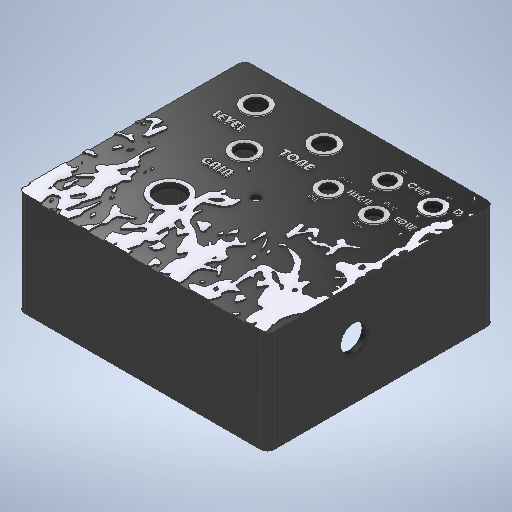
# Autodesk Inventor part: obudowa
Saved by Autodesk Inventor 2025 (Build 290162000, 162)
## iProperties
Created: 2026-04-02
Part Number: obudowa
Material: Ogólny
Document SubType Name: Modeling
Designer: zzapa
Density: 1 g/cm^3
Appearance: Domyślna
Author: zzapa
Autodesk Inventor part; units mm, degrees
(part 1 of 5)
ref_plane "YZ Plane" through (0, 0, 0) normal (1, 0, 0) x (0, 1, 0)
ref_plane "XZ Plane" through (0, 0, 0) normal (0, 1, 0) x (-1, 0, 0)
ref_plane "XY Plane" through (0, 0, 0) normal (0, 0, 1) x (1, 0, 0)
sketch "Szkic1" plane through (0, 0, 0) normal (0, 1, 0) x (-1, 0, 0)
  line L0 (110, -100) -> (0, -100)
  line L1 (0, -100) -> (0, 0)
  line L2 (0, 0) -> (110, 0)
  line L3 (110, 0) -> (110, -100)
  dimension "d0" = 100
  dimension "d1" = 110
  constraints: 8 end point, 2 parallel, 1 coincident, 1 horizontal, 1 perpendicular
  measures "d0" distance of L2.end L0.start
  measures "d1" distance of L0.start L0.end
extrude "Gabaryt" add sketch "Szkic1" along normal blind 45
ref_plane "Konstrukcja wycięcia" through (0, 43, 0) normal (0, 1, 0) x (1, 0, 0)
sketch "Szkic2" plane through (0, 0, 0) normal (0, -1, 0) x (1, 0, 0)
  line L0 (-110, 0) -> (0, 0) projected
  line L1 (-110, -100) -> (-110, 0) projected
  line L2 (0, -100) -> (-110, -100) projected
  line L3 (0, 0) -> (0, -100) projected
  line L4 (-2, -98) -> (-108, -98)
  line L5 (-108, -98) -> (-108, -2)
  line L6 (-108, -2) -> (-2, -2)
  line L7 (-2, -2) -> (-2, -98)
  dimension "d4" = 2
  constraints: 8 end point, 3 other
  measures "d4" distance between parallel lines of L3 L7
extrude "Wydrążenie" cut sketch "Szkic2" against normal up to surface (43 mm away) contours L4 L5 L6 L7
sketch "Szkic6" plane through (0, 0, 0) normal (0, -1, 0) x (1, 0, 0)
  line L0 (-110, 0) -> (0, 0) projected
  line L1 (-8, -8) -> (0, -8)
  line L2 (0, -8) -> (0, 0)
  line L3 (0, 0) -> (-8, 0)
  line L4 (-8, 0) -> (-8, -8)
  line L5 (0, 0) -> (0, -100) projected
  line L6 (0, -100) -> (-110, -100) projected
  line L7 (-110, -100) -> (-110, 0) projected
  line L8 (0, 0) -> (0, -100) projected
  line L9 (0, -50) -> (-110, -50)
  line L10 (-55, 0) -> (-55, -100)
  line L11 (-102, -8) -> (-110, -8)
  line L12 (-110, -8) -> (-110, 0)
  line L13 (-110, 0) -> (-102, 0)
  line L14 (-102, 0) -> (-102, -8)
  line L15 (-8, -92) -> (0, -92)
  line L16 (0, -92) -> (0, -100)
  line L17 (0, -100) -> (-8, -100)
  line L18 (-8, -100) -> (-8, -92)
  line L19 (-102, -92) -> (-110, -92)
  line L20 (-110, -92) -> (-110, -100)
  line L21 (-110, -100) -> (-102, -100)
  line L22 (-102, -100) -> (-102, -92)
  point P0 (-102, -100)
  point P1 (-110, -92)
  point P2 (-102, 0)
  point P3 (-8, -100)
  point P4 (0, -92)
  point P5 (-8, 0)
  dimension "d16" = 8
  dimension "d17" = 8
  constraints: 36 end point, 9 symmetric about line, 4 midpoint, 2 parallel, 1 horizontal, 1 perpendicular
  measures "d16" distance of L1.start L1.end
  measures "d17" distance of L3.end L1.start
extrude "Materiał na insert" add sketch "Szkic6" against normal up to surface (43 mm away) contours L0 L14 L11 L7 | L0 L2 L1 L4 | L19 L22 L6 L7 | L5 L6 L18 L15
sketch "Szkic7" plane through (0, 0, 0) normal (0, -1, 0) x (1, 0, 0)
  line L0 (0, 0) -> (0, -100) projected
  line L1 (0, -50) -> (-110, -50)
  line L2 (-110, -100) -> (-110, 0) projected
  line L3 (0, -100) -> (-110, -100) projected
  line L4 (-55, -100) -> (-55, 0)
  line L5 (-110, 0) -> (0, 0) projected
  point P0 (-4, -4)
  point P1 (-106, -4)
  point P2 (-4, -96)
  point P3 (-106, -96)
  dimension "d20" = 4
  dimension "d21" = 4
  constraints: 4 end point, 4 midpoint, 3 symmetric about line
  measures "d20" horizontal distance of L0.start point (-4, -4)
  measures "d21" horizontal distance of point (-4, -4) L0.start
hole "Otwory montażowe" at (-4, 0, -4) at (-106, 0, -4) at (-4, 0, -96) at (-106, 0, -96) direction (0, 1, 0) diameter 2.4 depth 5.5
fillet "Zaokrąglenie1" radius 3 4 edges at (-110, 22.5, 0) (0, 22.5, 0) (0, 22.5, -100) (-110, 22.5, -100)
sketch "Szkic8" plane through (-110, 0, -97) normal (-1, 0, 0) x (0, 0, 1)
  line L0 (-3, 45) -> (-3, 0) projected
  line L1 (0, 0) -> (94, 0) projected
  line L2 (0, 0) -> (-3, 0) projected
  line L3 (97, 0) -> (97, 45) projected
  point P0 (42, 25)
  dimension "d30" = 25
  dimension "d39" = 55
  measures "d30" distance from line of L1 point (42, 25)
  measures "d39" distance from line of L3 point (42, 25)
hole "JACK 1" at (-110, 25, -55) direction (1, 0, 0) diameter 11.5 depth 2
sketch "Szkic9" plane through (0, 0, -3) normal (1, 0, 0) x (0, 0, -1)
  line L0 (0, 0) -> (94, 0) projected
  line L1 (-3, 45) -> (-3, 0) projected
  point P0 (35, 25)
  dimension "d40" = 25
  dimension "d41" = 38
  measures "d40" distance from line of L0 point (35, 25)
  measures "d41" distance from line of point (35, 25) L1
hole "JACK 2" at (0, 25, -38) direction (-1, 0, 0) diameter 11.5 end up to face face through (-2, 14.3333, -64) facing (-1, 0, 0)
sketch "Szkic16" plane through (0, 45, 0) normal (0, 1, 0) x (1, 0, 0)
  line L0 (-138.1067, 105.9838) -> (23.8181, 105.9838)
  line L1 (23.8181, 105.9838) -> (23.8181, 34.811)
  line L2 (23.8181, 34.811) -> (23.0109, 35.22)
  line L3 (23.0109, 35.22) -> (22.3629, 35.8693)
  line L4 (22.3629, 35.8693) -> (21.7155, 38.0761)
  line L5 (21.7155, 38.0761) -> (20.9077, 40.2349)
  line L6 (20.9077, 40.2349) -> (21.2638, 40.857)
  line L7 (21.2638, 40.857) -> (21.4369, 41.5579)
  line L8 (21.4369, 41.5579) -> (21.3046, 46.1881)
  line L9 (21.3046, 46.1881) -> (20.2689, 48.7465)
  line L10 (20.2689, 48.7465) -> (19.0556, 51.2151)
  line L11 (19.0556, 51.2151) -> (19.3469, 52.5366)
  line L12 (19.3469, 52.5366) -> (19.4525, 53.861)
  line L13 (19.4525, 53.861) -> (19.1879, 54.3901)
  line L14 (19.1879, 54.3901) -> (18.0583, 53.9543)
  line L15 (18.0583, 53.9543) -> (17.1306, 54.0295)
  line L16 (17.1306, 54.0295) -> (16.4047, 54.6158)
  line L17 (16.4047, 54.6158) -> (15.8806, 55.7131)
  line L18 (15.8806, 55.7131) -> (16.2764, 57.0344)
  line L19 (16.2764, 57.0344) -> (16.939, 58.2266)
  line L20 (16.939, 58.2266) -> (19.3202, 58.6235)
  line L21 (19.3202, 58.6235) -> (19.5271, 59.3328)
  line L22 (19.5271, 59.3328) -> (19.53, 60.0102)
  line L23 (19.53, 60.0102) -> (19.3287, 60.6557)
  line L24 (19.3287, 60.6557) -> (18.9233, 61.2693)
  line L25 (18.9233, 61.2693) -> (17.8565, 60.6698)
  line L26 (17.8565, 60.6698) -> (16.6744, 60.3433)
  line L27 (16.6744, 60.3433) -> (16.2775, 58.6235)
  line L28 (16.2775, 58.6235) -> (15.4838, 58.0943)
  line L29 (15.4838, 58.0943) -> (15.0261, 58.2056)
  line L30 (15.0261, 58.2056) -> (14.631, 58.1325)
  line L31 (14.631, 58.1325) -> (14.2984, 57.8749)
  line L32 (14.2984, 57.8749) -> (14.0286, 57.4328)
  line L33 (14.0286, 57.4328) -> (12.4411, 57.3005)
  line L34 (12.4411, 57.3005) -> (10.8536, 57.4328)
  line L35 (10.8536, 57.4328) -> (9.5248, 58.7629)
  line L36 (9.5248, 58.7629) -> (8.4723, 60.3433)
  line L37 (8.4723, 60.3433) -> (1.4609, 64.1797)
  line L38 (1.4609, 64.1797) -> (-0.1266, 67.3547)
  line L39 (-0.1266, 67.3547) -> (-0.1433, 69.3393)
  line L40 (-0.1433, 69.3393) -> (0.0057, 71.3234)
  line L41 (0.0057, 71.3234) -> (-0.7881, 71.3234)
  line L42 (-0.7881, 71.3234) -> (-1.1487, 69.1464)
  line L43 (-1.1487, 69.1464) -> (-1.3629, 68.6021)
  line L44 (-1.3629, 68.6021) -> (-1.5997, 68.4207)
  line L45 (-1.5997, 68.4207) -> (-1.859, 68.6021)
  line L46 (-1.859, 68.6021) -> (-2.1409, 69.1464)
  line L47 (-2.1409, 69.1464) -> (-2.7725, 71.3234)
  line L48 (-2.7725, 71.3234) -> (-2.9048, 72.7787)
  line L49 (-2.9048, 72.7787) -> (-2.7725, 74.2339)
  line L50 (-2.7725, 74.2339) -> (2.1223, 76.4828)
  line L51 (2.1223, 76.4828) -> (3.588, 77.6838)
  line L52 (3.588, 77.6838) -> (4.6359, 79.2609)
  line L53 (4.6359, 79.2609) -> (4.7682, 81.6422)
  line L54 (4.7682, 81.6422) -> (4.6359, 84.0234)
  line L55 (4.6359, 84.0234) -> (3.1196, 87.6571)
  line L56 (3.1196, 87.6571) -> (1.3286, 91.1672)
  line L57 (1.3286, 91.1672) -> (0.4638, 91.3959)
  line L58 (0.4638, 91.3959) -> (-0.2654, 91.2958)
  line L59 (-0.2654, 91.2958) -> (-0.8591, 90.8667)
  line L60 (-0.8591, 90.8667) -> (-1.3173, 90.1088)
  line L61 (-1.3173, 90.1088) -> (-0.6682, 89.4152)
  line L62 (-0.6682, 89.4152) -> (0.2702, 89.1828)
  line L63 (0.2702, 89.1828) -> (0.7636, 88.4018)
  line L64 (0.7636, 88.4018) -> (1.1044, 87.5683)
  line L65 (1.1044, 87.5683) -> (1.2928, 86.682)
  line L66 (1.2928, 86.682) -> (1.3286, 85.7432)
  line L67 (1.3286, 85.7432) -> (1.1916, 84.5366)
  line L68 (1.1916, 84.5366) -> (0.9519, 83.618)
  line L69 (0.9519, 83.618) -> (0.6097, 82.9875)
  line L70 (0.6097, 82.9875) -> (0.1649, 82.645)
  line L71 (0.1649, 82.645) -> (-0.3824, 82.5906)
  line L72 (-0.3824, 82.5906) -> (-1.0324, 82.8243)
  line L73 (-1.0324, 82.8243) -> (-1.785, 83.346)
  line L74 (-1.785, 83.346) -> (-2.6402, 84.1557)
  line L75 (-2.6402, 84.1557) -> (-3.4339, 84.288)
  line L76 (-3.4339, 84.288) -> (-3.408, 82.9177)
  line L77 (-3.408, 82.9177) -> (-3.7742, 81.7554)
  line L78 (-3.7742, 81.7554) -> (-4.5325, 80.8011)
  line L79 (-4.5325, 80.8011) -> (-5.6829, 80.0547)
  line L80 (-5.6829, 80.0547) -> (-5.9576, 79.4144)
  line L81 (-5.9576, 79.4144) -> (-6.0271, 78.782)
  line L82 (-6.0271, 78.782) -> (-5.8915, 78.1577)
  line L83 (-5.8915, 78.1577) -> (-5.5506, 77.5411)
  line L84 (-5.5506, 77.5411) -> (-6.0348, 75.915)
  line L85 (-6.0348, 75.915) -> (-6.3443, 74.2339)
  line L86 (-6.3443, 74.2339) -> (-6.0798, 72.9109)
  line L87 (-6.0798, 72.9109) -> (-6.3443, 71.588)
  line L88 (-6.3443, 71.588) -> (-3.1693, 63.7828)
  line L89 (-3.1693, 63.7828) -> (-3.5662, 62.3276)
  line L90 (-3.5662, 62.3276) -> (-4.1521, 61.7435)
  line L91 (-4.1521, 61.7435) -> (-4.4922, 61.0047)
  line L92 (-4.4922, 61.0047) -> (-3.5983, 56.4054)
  line L93 (-3.5983, 56.4054) -> (-3.3753, 54.0825)
  line L94 (-3.3753, 54.0825) -> (-3.3016, 51.7443)
  line L95 (-3.3016, 51.7443) -> (-4.0954, 50.1568)
  line L96 (-4.0954, 50.1568) -> (-7.0058, 47.7756)
  line L97 (-7.0058, 47.7756) -> (-7.535, 45.3943)
  line L98 (-7.535, 45.3943) -> (-9.1611, 44.8525)
  line L99 (-9.1611, 44.8525) -> (-10.8422, 44.4683)
  line L100 (-10.8422, 44.4683) -> (-11.3602, 43.7585)
  line L101 (-11.3602, 43.7585) -> (-11.6431, 43.0148)
  line L102 (-11.6431, 43.0148) -> (-11.6909, 42.2371)
  line L103 (-11.6909, 42.2371) -> (-11.5037, 41.4256)
  line L104 (-11.5037, 41.4256) -> (-10.3341, 40.2553)
  line L105 (-10.3341, 40.2553) -> (-8.9902, 39.3089)
  line L106 (-8.9902, 39.3089) -> (-8.0825, 39.6923)
  line L107 (-8.0825, 39.6923) -> (-7.1846, 39.8201)
  line L108 (-7.1846, 39.8201) -> (-6.2965, 39.6923)
  line L109 (-6.2965, 39.6923) -> (-5.4183, 39.3089)
  line L110 (-5.4183, 39.3089) -> (-5.1545, 38.9347)
  line L111 (-5.1545, 38.9347) -> (-5.0887, 38.5675)
  line L112 (-5.0887, 38.5675) -> (-5.2207, 38.2072)
  line L113 (-5.2207, 38.2072) -> (-5.5506, 37.8537)
  line L114 (-5.5506, 37.8537) -> (-6.457, 37.4644)
  line L115 (-6.457, 37.4644) -> (-7.2704, 36.9277)
  line L116 (-7.2704, 36.9277) -> (-7.3598, 36.574)
  line L117 (-7.3598, 36.574) -> (-7.1381, 36.2662)
  line L118 (-7.1381, 36.2662) -> (-6.6089, 36.1338)
  line L119 (-6.6089, 36.1338) -> (-6.0797, 36.2662)
  line L120 (-6.0797, 36.2662) -> (-5.3543, 36.8938)
  line L121 (-5.3543, 36.8938) -> (-4.4922, 37.3245)
  line L122 (-4.4922, 37.3245) -> (-4.2715, 38.0841)
  line L123 (-4.2715, 38.0841) -> (-4.2277, 38.7797)
  line L124 (-4.2277, 38.7797) -> (-2.6402, 37.7214)
  line L125 (-2.6402, 37.7214) -> (-2.0611, 35.7499)
  line L126 (-2.0611, 35.7499) -> (-1.7141, 33.7527)
  line L127 (-1.7141, 33.7527) -> (-2.2126, 34.1473)
  line L128 (-2.2126, 34.1473) -> (-2.6654, 34.2568)
  line L129 (-2.6654, 34.2568) -> (-3.0725, 34.0812)
  line L130 (-3.0725, 34.0812) -> (-3.4339, 33.6204)
  line L131 (-3.4339, 33.6204) -> (-3.1209, 33.0089)
  line L132 (-3.1209, 33.0089) -> (-2.7299, 32.7389)
  line L133 (-2.7299, 32.7389) -> (-2.261, 32.8104)
  line L134 (-2.261, 32.8104) -> (-1.7141, 33.2235)
  line L135 (-1.7141, 33.2235) -> (-1.4495, 32.9589)
  line L136 (-1.4495, 32.9589) -> (-1.7141, 30.0485)
  line L137 (-1.7141, 30.0485) -> (-0.1266, 29.2548)
  line L138 (-0.1266, 29.2548) -> (0.0057, 28.461)
  line L139 (0.0057, 28.461) -> (-0.1266, 27.6673)
  line L140 (-0.1266, 27.6673) -> (-1.9787, 27.4027)
  line L141 (-1.9787, 27.4027) -> (-2.4802, 26.1616)
  line L142 (-2.4802, 26.1616) -> (-3.1693, 25.0214)
  line L143 (-3.1693, 25.0214) -> (-2.9048, 24.4923)
  line L144 (-2.9048, 24.4923) -> (-3.1693, 23.9631)
  line L145 (-3.1693, 23.9631) -> (-6.0797, 23.8308)
  line L146 (-6.0797, 23.8308) -> (-6.6591, 23.3711)
  line L147 (-6.6591, 23.3711) -> (-7.2491, 23.2178)
  line L148 (-7.2491, 23.2178) -> (-7.8498, 23.3711)
  line L149 (-7.8498, 23.3711) -> (-8.461, 23.8308)
  line L150 (-8.461, 23.8308) -> (-9.1787, 24.6043)
  line L151 (-9.1787, 24.6043) -> (-9.6516, 25.5506)
  line L152 (-9.6516, 25.5506) -> (-10.0048, 27.4854)
  line L153 (-10.0048, 27.4854) -> (-10.0485, 29.387)
  line L154 (-10.0485, 29.387) -> (-10.9894, 29.4565)
  line L155 (-10.9894, 29.4565) -> (-11.6999, 29.1931)
  line L156 (-11.6999, 29.1931) -> (-12.18, 28.5967)
  line L157 (-12.18, 28.5967) -> (-12.4297, 27.6673)
  line L158 (-12.4297, 27.6673) -> (-12.8266, 27.2703)
  line L159 (-12.8266, 27.2703) -> (-13.2235, 27.138)
  line L160 (-13.2235, 27.138) -> (-13.6204, 27.2703)
  line L161 (-13.6204, 27.2703) -> (-14.0172, 27.6673)
  line L162 (-14.0172, 27.6673) -> (-15.0756, 29.387)
  line L163 (-15.0756, 29.387) -> (-15.8613, 29.6807)
  line L164 (-15.8613, 29.6807) -> (-16.4539, 30.1534)
  line L165 (-16.4539, 30.1534) -> (-16.8535, 30.8052)
  line L166 (-16.8535, 30.8052) -> (-17.0599, 31.636)
  line L167 (-17.0599, 31.636) -> (-20.8964, 36.0016)
  line L168 (-20.8964, 36.0016) -> (-25.3943, 37.3245)
  line L169 (-25.3943, 37.3245) -> (-26.8515, 37.5331)
  line L170 (-26.8515, 37.5331) -> (-28.3047, 37.5891)
  line L171 (-28.3047, 37.5891) -> (-28.5692, 37.3245)
  line L172 (-28.5692, 37.3245) -> (-28.3047, 37.06)
  line L173 (-28.3047, 37.06) -> (-24.5793, 35.33)
  line L174 (-24.5793, 35.33) -> (-21.161, 33.0912)
  line L175 (-21.161, 33.0912) -> (-19.5551, 30.806)
  line L176 (-19.5551, 30.806) -> (-18.2506, 28.3287)
  line L177 (-18.2506, 28.3287) -> (-19.1787, 27.2531)
  line L178 (-19.1787, 27.2531) -> (-20.2818, 26.5197)
  line L179 (-20.2818, 26.5197) -> (-21.5599, 26.1286)
  line L180 (-21.5599, 26.1286) -> (-23.0131, 26.0798)
  line L181 (-23.0131, 26.0798) -> (-25.1306, 26.2504)
  line L182 (-25.1306, 26.2504) -> (-27.2464, 25.9475)
  line L183 (-27.2464, 25.9475) -> (-27.6953, 25.1448)
  line L184 (-27.6953, 25.1448) -> (-27.889, 24.3261)
  line L185 (-27.889, 24.3261) -> (-27.8275, 23.4912)
  line L186 (-27.8275, 23.4912) -> (-27.511, 22.6402)
  line L187 (-27.511, 22.6402) -> (-28.3047, 20.3912)
  line L188 (-28.3047, 20.3912) -> (-27.2464, 13.2475)
  line L189 (-27.2464, 13.2475) -> (-27.511, 11.66)
  line L190 (-27.511, 11.66) -> (-27.7756, 11.5277)
  line L191 (-27.7756, 11.5277) -> (-28.0306, 12.165)
  line L192 (-28.0306, 12.165) -> (-28.0401, 12.8506)
  line L193 (-28.0401, 12.8506) -> (-28.8807, 12.6734)
  line L194 (-28.8807, 12.6734) -> (-29.4953, 12.0569)
  line L195 (-29.4953, 12.0569) -> (-30.8183, 9.6756)
  line L196 (-30.8183, 9.6756) -> (-31.612, 4.6485)
  line L197 (-31.612, 4.6485) -> (-32.2735, 3.9871)
  line L198 (-32.2735, 3.9871) -> (-34.1565, 3.5577)
  line L199 (-34.1565, 3.5577) -> (-35.9776, 2.9287)
  line L200 (-35.9776, 2.9287) -> (-36.2243, 2.2225)
  line L201 (-36.2243, 2.2225) -> (-36.1099, 1.4735)
  line L202 (-36.1099, 1.4735) -> (-34.1255, -0.2463)
  line L203 (-34.1255, -0.2463) -> (-31.4797, -0.2463)
  line L204 (-31.4797, -0.2463) -> (-30.7853, -1.0092)
  line L205 (-30.7853, -1.0092) -> (-30.4214, -1.966)
  line L206 (-30.4214, -1.966) -> (-39.1526, -1.966)
  line L207 (-39.1526, -1.966) -> (-38.8027, 0.0962)
  line L208 (-38.8027, 0.0962) -> (-38.7963, 2.1506)
  line L209 (-38.7963, 2.1506) -> (-39.1334, 4.1972)
  line L210 (-39.1334, 4.1972) -> (-39.8141, 6.236)
  line L211 (-39.8141, 6.236) -> (-39.9464, 7.8235)
  line L212 (-39.9464, 7.8235) -> (-39.8141, 9.411)
  line L213 (-39.8141, 9.411) -> (-39.4254, 10.189)
  line L214 (-39.4254, 10.189) -> (-38.888, 10.8662)
  line L215 (-38.888, 10.8662) -> (-37.0454, 11.9188)
  line L216 (-37.0454, 11.9188) -> (-35.3162, 13.1152)
  line L217 (-35.3162, 13.1152) -> (-34.2564, 12.3146)
  line L218 (-34.2564, 12.3146) -> (-33.4641, 11.2631)
  line L219 (-33.4641, 11.2631) -> (-33.0886, 11.3881)
  line L220 (-33.0886, 11.3881) -> (-32.8026, 11.66)
  line L221 (-32.8026, 11.66) -> (-34.1364, 13.789)
  line L222 (-34.1364, 13.789) -> (-35.713, 15.761)
  line L223 (-35.713, 15.761) -> (-36.9086, 16.0817)
  line L224 (-36.9086, 16.0817) -> (-38.0943, 16.0256)
  line L225 (-38.0943, 16.0256) -> (-37.3997, 15.6813)
  line L226 (-37.3997, 15.6813) -> (-36.8815, 15.2137)
  line L227 (-36.8815, 15.2137) -> (-36.5397, 14.623)
  line L228 (-36.5397, 14.623) -> (-36.3745, 13.9089)
  line L229 (-36.3745, 13.9089) -> (-36.906, 13.4522)
  line L230 (-36.906, 13.4522) -> (-37.48, 13.2118)
  line L231 (-37.48, 13.2118) -> (-38.0966, 13.1876)
  line L232 (-38.0966, 13.1876) -> (-38.7557, 13.3798)
  line L233 (-38.7557, 13.3798) -> (-39.4851, 12.7013)
  line L234 (-39.4851, 12.7013) -> (-40.4755, 12.586)
  line L235 (-40.4755, 12.586) -> (-40.2419, 14.0455)
  line L236 (-40.2419, 14.0455) -> (-39.7451, 15.3698)
  line L237 (-39.7451, 15.3698) -> (-38.9851, 16.5591)
  line L238 (-38.9851, 16.5591) -> (-37.962, 17.6131)
  line L239 (-37.962, 17.6131) -> (-37.5934, 19.1841)
  line L240 (-37.5934, 19.1841) -> (-37.8297, 20.7881)
  line L241 (-37.8297, 20.7881) -> (-39.4129, 21.5569)
  line L242 (-39.4129, 21.5569) -> (-40.5863, 22.3706)
  line L243 (-40.5863, 22.3706) -> (-41.3499, 23.2292)
  line L244 (-41.3499, 23.2292) -> (-41.7036, 24.1328)
  line L245 (-41.7036, 24.1328) -> (-41.6475, 25.0813)
  line L246 (-41.6475, 25.0813) -> (-41.1816, 26.0747)
  line L247 (-41.1816, 26.0747) -> (-40.3059, 27.1131)
  line L248 (-40.3059, 27.1131) -> (-39.0203, 28.1964)
  line L249 (-39.0203, 28.1964) -> (-38.6861, 29.0417)
  line L250 (-38.6861, 29.0417) -> (-38.729, 29.6982)
  line L251 (-38.729, 29.6982) -> (-39.1491, 30.1661)
  line L252 (-39.1491, 30.1661) -> (-39.9464, 30.4454)
  line L253 (-39.9464, 30.4454) -> (-40.3009, 29.6426)
  line L254 (-40.3009, 29.6426) -> (-40.8724, 28.9902)
  line L255 (-40.8724, 28.9902) -> (-41.9146, 29.5033)
  line L256 (-41.9146, 29.5033) -> (-42.8568, 30.1808)
  line L257 (-42.8568, 30.1808) -> (-43.5366, 30.306)
  line L258 (-43.5366, 30.306) -> (-44.1797, 30.0485)
  line L259 (-44.1797, 30.0485) -> (-43.2841, 28.6643)
  line L260 (-43.2841, 28.6643) -> (-43.1264, 28.0537)
  line L261 (-43.1264, 28.0537) -> (-43.162, 27.4974)
  line L262 (-43.162, 27.4974) -> (-43.391, 26.9954)
  line L263 (-43.391, 26.9954) -> (-43.8134, 26.5477)
  line L264 (-43.8134, 26.5477) -> (-45.238, 25.8152)
  line L265 (-45.238, 25.8152) -> (-45.8113, 25.9916)
  line L266 (-45.8113, 25.9916) -> (-46.2964, 26.3443)
  line L267 (-46.2964, 26.3443) -> (-46.8255, 25.5506)
  line L268 (-46.8255, 25.5506) -> (-45.7672, 22.5079)
  line L269 (-45.7672, 22.5079) -> (-45.9219, 22.0886)
  line L270 (-45.9219, 22.0886) -> (-46.2964, 21.8464)
  line L271 (-46.2964, 21.8464) -> (-47.7516, 22.9048)
  line L272 (-47.7516, 22.9048) -> (-48.1484, 22.5079)
  line L273 (-48.1484, 22.5079) -> (-46.8255, 20.7881)
  line L274 (-46.8255, 20.7881) -> (-47.3547, 19.4652)
  line L275 (-47.3547, 19.4652) -> (-48.9521, 19.2457)
  line L276 (-48.9521, 19.2457) -> (-50.5297, 19.5975)
  line L277 (-50.5297, 19.5975) -> (-51.946, 21.0018)
  line L278 (-51.946, 21.0018) -> (-53.4765, 22.2637)
  line L279 (-53.4765, 22.2637) -> (-55.121, 23.3831)
  line L280 (-55.121, 23.3831) -> (-56.8797, 24.36)
  line L281 (-56.8797, 24.36) -> (-58.39, 24.9104)
  line L282 (-58.39, 24.9104) -> (-59.6211, 25.7774)
  line L283 (-59.6211, 25.7774) -> (-60.5728, 26.9609)
  line L284 (-60.5728, 26.9609) -> (-61.2453, 28.461)
  line L285 (-61.2453, 28.461) -> (-61.5301, 29.4351)
  line L286 (-61.5301, 29.4351) -> (-61.6422, 30.4454)
  line L287 (-61.6422, 30.4454) -> (-61.4954, 31.704)
  line L288 (-61.4954, 31.704) -> (-61.5099, 32.9589)
  line L289 (-61.5099, 32.9589) -> (-61.9068, 33.2235)
  line L290 (-61.9068, 33.2235) -> (-62.9651, 30.3131)
  line L291 (-62.9651, 30.3131) -> (-63.7676, 31.5253)
  line L292 (-63.7676, 31.5253) -> (-64.1557, 32.9589)
  line L293 (-64.1557, 32.9589) -> (-64.3891, 34.5696)
  line L294 (-64.3891, 34.5696) -> (-64.1557, 36.1339)
  line L295 (-64.1557, 36.1339) -> (-59.2609, 38.3829)
  line L296 (-59.2609, 38.3829) -> (-58.2504, 39.0964)
  line L297 (-58.2504, 39.0964) -> (-57.4726, 39.9737)
  line L298 (-57.4726, 39.9737) -> (-56.9275, 41.0147)
  line L299 (-56.9275, 41.0147) -> (-56.6151, 42.2193)
  line L300 (-56.6151, 42.2193) -> (-56.7474, 45.1297)
  line L301 (-56.7474, 45.1297) -> (-57.3205, 45.3719)
  line L302 (-57.3205, 45.3719) -> (-57.938, 45.262)
  line L303 (-57.938, 45.262) -> (-58.6076, 44.4039)
  line L304 (-58.6076, 44.4039) -> (-59.4041, 43.9194)
  line L305 (-59.4041, 43.9194) -> (-60.3274, 43.8086)
  line L306 (-60.3274, 43.8086) -> (-61.3776, 44.0714)
  line L307 (-61.3776, 44.0714) -> (-62.4004, 43.6928)
  line L308 (-62.4004, 43.6928) -> (-63.2297, 43.0131)
  line L309 (-63.2297, 43.0131) -> (-63.4943, 43.2777)
  line L310 (-63.4943, 43.2777) -> (-63.1209, 43.7814)
  line L311 (-63.1209, 43.7814) -> (-62.9744, 44.3021)
  line L312 (-62.9744, 44.3021) -> (-63.0547, 44.8397)
  line L313 (-63.0547, 44.8397) -> (-63.362, 45.3943)
  line L314 (-63.362, 45.3943) -> (-64.0124, 45.8551)
  line L315 (-64.0124, 45.8551) -> (-64.8172, 45.9235)
  line L316 (-64.8172, 45.9235) -> (-64.9495, 44.0714)
  line L317 (-64.9495, 44.0714) -> (-67.0661, 41.4256)
  line L318 (-67.0661, 41.4256) -> (-67.7276, 35.2079)
  line L319 (-67.7276, 35.2079) -> (-67.5953, 32.4297)
  line L320 (-67.5953, 32.4297) -> (-66.4892, 30.4341)
  line L321 (-66.4892, 30.4341) -> (-65.6109, 28.3287)
  line L322 (-65.6109, 28.3287) -> (-65.8969, 28.0569)
  line L323 (-65.8969, 28.0569) -> (-66.2724, 27.9318)
  line L324 (-66.2724, 27.9318) -> (-68.0585, 28.7584)
  line L325 (-68.0585, 28.7584) -> (-69.712, 29.7839)
  line L326 (-69.712, 29.7839) -> (-70.5057, 32.9589)
  line L327 (-70.5057, 32.9589) -> (-70.7581, 32.4963)
  line L328 (-70.7581, 32.4963) -> (-70.8202, 32.0334)
  line L329 (-70.8202, 32.0334) -> (-70.692, 31.5702)
  line L330 (-70.692, 31.5702) -> (-70.3734, 31.1068)
  line L331 (-70.3734, 31.1068) -> (-70.563, 30.1469)
  line L332 (-70.563, 30.1469) -> (-70.979, 29.364)
  line L333 (-70.979, 29.364) -> (-71.6214, 28.7579)
  line L334 (-71.6214, 28.7579) -> (-72.4901, 28.3287)
  line L335 (-72.4901, 28.3287) -> (-73.6247, 27.1948)
  line L336 (-73.6247, 27.1948) -> (-74.6067, 25.9475)
  line L337 (-74.6067, 25.9475) -> (-74.2868, 25.3081)
  line L338 (-74.2868, 25.3081) -> (-74.136, 24.6539)
  line L339 (-74.136, 24.6539) -> (-74.1545, 23.9851)
  line L340 (-74.1545, 23.9851) -> (-74.3422, 23.3016)
  line L341 (-74.3422, 23.3016) -> (-74.0142, 22.7184)
  line L342 (-74.0142, 22.7184) -> (-73.5961, 22.4358)
  line L343 (-73.5961, 22.4358) -> (-73.0881, 22.4538)
  line L344 (-73.0881, 22.4538) -> (-72.4901, 22.7725)
  line L345 (-72.4901, 22.7725) -> (-70.846, 24.1135)
  line L346 (-70.846, 24.1135) -> (-70.2283, 24.3413)
  line L347 (-70.2283, 24.3413) -> (-69.7468, 24.2739)
  line L348 (-69.7468, 24.2739) -> (-69.4015, 23.9113)
  line L349 (-69.4015, 23.9113) -> (-69.1924, 23.2536)
  line L350 (-69.1924, 23.2536) -> (-69.1828, 21.0527)
  line L351 (-69.1828, 21.0527) -> (-67.9922, 17.3485)
  line L352 (-67.9922, 17.3485) -> (-68.0951, 16.9229)
  line L353 (-68.0951, 16.9229) -> (-68.3057, 16.6708)
  line L354 (-68.3057, 16.6708) -> (-68.6242, 16.5922)
  line L355 (-68.6242, 16.5922) -> (-69.0505, 16.6871)
  line L356 (-69.0505, 16.6871) -> (-69.8572, 18.8427)
  line L357 (-69.8572, 18.8427) -> (-70.5057, 21.0527)
  line L358 (-70.5057, 21.0527) -> (-71.2849, 21.0981)
  line L359 (-71.2849, 21.0981) -> (-71.7652, 20.8487)
  line L360 (-71.7652, 20.8487) -> (-71.9464, 20.3044)
  line L361 (-71.9464, 20.3044) -> (-71.8286, 19.4652)
  line L362 (-71.8286, 19.4652) -> (-70.7346, 17.8066)
  line L363 (-70.7346, 17.8066) -> (-69.4474, 16.2902)
  line L364 (-69.4474, 16.2902) -> (-69.3348, 15.2084)
  line L365 (-69.3348, 15.2084) -> (-69.5398, 14.2524)
  line L366 (-69.5398, 14.2524) -> (-70.0624, 13.4224)
  line L367 (-70.0624, 13.4224) -> (-70.9026, 12.7183)
  line L368 (-70.9026, 12.7183) -> (-72.1541, 12.3764)
  line L369 (-72.1541, 12.3764) -> (-73.4161, 12.3214)
  line L370 (-73.4161, 12.3214) -> (-73.4655, 11.1487)
  line L371 (-73.4655, 11.1487) -> (-73.3496, 10.0081)
  line L372 (-73.3496, 10.0081) -> (-73.0686, 8.8997)
  line L373 (-73.0686, 8.8997) -> (-72.6224, 7.8235)
  line L374 (-72.6224, 7.8235) -> (-71.197, 8.9175)
  line L375 (-71.197, 8.9175) -> (-69.9943, 10.1862)
  line L376 (-69.9943, 10.1862) -> (-69.0142, 11.6295)
  line L377 (-69.0142, 11.6295) -> (-68.2568, 13.2475)
  line L378 (-68.2568, 13.2475) -> (-67.4827, 13.5231)
  line L379 (-67.4827, 13.5231) -> (-66.8278, 13.4606)
  line L380 (-66.8278, 13.4606) -> (-66.2921, 13.0601)
  line L381 (-66.2921, 13.0601) -> (-65.8755, 12.3214)
  line L382 (-65.8755, 12.3214) -> (-66.4047, 11.3954)
  line L383 (-66.4047, 11.3954) -> (-67.6284, 10.6671)
  line L384 (-67.6284, 10.6671) -> (-68.4552, 9.6968)
  line L385 (-68.4552, 9.6968) -> (-68.8851, 8.4843)
  line L386 (-68.8851, 8.4843) -> (-68.9182, 7.0298)
  line L387 (-68.9182, 7.0298) -> (-69.8443, 6.1037)
  line L388 (-69.8443, 6.1037) -> (-73.1515, 4.9131)
  line L389 (-73.1515, 4.9131) -> (-72.6447, 2.0679)
  line L390 (-72.6447, 2.0679) -> (-71.564, -0.6431)
  line L391 (-71.564, -0.6431) -> (-71.4317, -1.966)
  line L392 (-71.4317, -1.966) -> (-78.3109, -1.966)
  line L393 (-78.3109, -1.966) -> (-78.6487, -0.117)
  line L394 (-78.6487, -0.117) -> (-78.7833, 1.7342)
  line L395 (-78.7833, 1.7342) -> (-78.7148, 3.5872)
  line L396 (-78.7148, 3.5872) -> (-78.4432, 5.4423)
  line L397 (-78.4432, 5.4423) -> (-77.5172, 7.0298)
  line L398 (-77.5172, 7.0298) -> (-77.9934, 9.3856)
  line L399 (-77.9934, 9.3856) -> (-77.914, 11.7923)
  line L400 (-77.914, 11.7923) -> (-75.9132, 13.1238)
  line L401 (-75.9132, 13.1238) -> (-73.813, 14.3058)
  line L402 (-73.813, 14.3058) -> (-73.3758, 14.8237)
  line L403 (-73.3758, 14.8237) -> (-73.2838, 15.4964)
  line L404 (-73.2838, 15.4964) -> (-78.1786, 13.9089)
  line L405 (-78.1786, 13.9089) -> (-79.1047, 14.0412)
  line L406 (-79.1047, 14.0412) -> (-79.8984, 15.3641)
  line L407 (-79.8984, 15.3641) -> (-81.421, 15.6178)
  line L408 (-81.421, 15.6178) -> (-82.8088, 16.2902)
  line L409 (-82.8088, 16.2902) -> (-83.0683, 15.5121)
  line L410 (-83.0683, 15.5121) -> (-82.9411, 14.7027)
  line L411 (-82.9411, 14.7027) -> (-81.6355, 12.3423)
  line L412 (-81.6355, 12.3423) -> (-80.0307, 10.2048)
  line L413 (-80.0307, 10.2048) -> (-79.6922, 8.0573)
  line L414 (-79.6922, 8.0573) -> (-79.1047, 5.9714)
  line L415 (-79.1047, 5.9714) -> (-79.3476, 4.6235)
  line L416 (-79.3476, 4.6235) -> (-79.7661, 3.3256)
  line L417 (-79.7661, 3.3256) -> (-81.454, 1.6399)
  line L418 (-81.454, 1.6399) -> (-82.6765, -0.3785)
  line L419 (-82.6765, -0.3785) -> (-82.8088, -1.966)
  line L420 (-82.8088, -1.966) -> (-88.1005, -1.966)
  line L421 (-88.1005, -1.966) -> (-87.5068, 1.3222)
  line L422 (-87.5068, 1.3222) -> (-86.513, 4.5162)
  line L423 (-86.513, 4.5162) -> (-87.1071, 5.8402)
  line L424 (-87.1071, 5.8402) -> (-87.3067, 7.2944)
  line L425 (-87.3067, 7.2944) -> (-86.9263, 10.5984)
  line L426 (-86.9263, 10.5984) -> (-87.0421, 13.9089)
  line L427 (-87.0421, 13.9089) -> (-87.439, 13.6444)
  line L428 (-87.439, 13.6444) -> (-88.0062, 10.279)
  line L429 (-88.0062, 10.279) -> (-89.0265, 7.0298)
  line L430 (-89.0265, 7.0298) -> (-90.0294, 5.553)
  line L431 (-90.0294, 5.553) -> (-90.614, 3.8548)
  line L432 (-90.614, 3.8548) -> (-91.2286, 3.2382)
  line L433 (-91.2286, 3.2382) -> (-92.0692, 3.061)
  line L434 (-92.0692, 3.061) -> (-91.4592, 5.8191)
  line L435 (-91.4592, 5.8191) -> (-91.0109, 8.6173)
  line L436 (-91.0109, 8.6173) -> (-91.2755, 9.2787)
  line L437 (-91.2755, 9.2787) -> (-89.1588, 15.761)
  line L438 (-89.1588, 15.761) -> (-90.4507, 18.0829)
  line L439 (-90.4507, 18.0829) -> (-91.2755, 20.6558)
  line L440 (-91.2755, 20.6558) -> (-90.7339, 22.0389)
  line L441 (-90.7339, 22.0389) -> (-90.399, 23.448)
  line L442 (-90.399, 23.448) -> (-90.2708, 24.8832)
  line L443 (-90.2708, 24.8832) -> (-90.3494, 26.3443)
  line L444 (-90.3494, 26.3443) -> (-89.4059, 27.4096)
  line L445 (-89.4059, 27.4096) -> (-88.6296, 28.5933)
  line L446 (-88.6296, 28.5933) -> (-89.2902, 29.4549)
  line L447 (-89.2902, 29.4549) -> (-90.2171, 30.0485)
  line L448 (-90.2171, 30.0485) -> (-90.8786, 33.4881)
  line L449 (-90.8786, 33.4881) -> (-91.5401, 33.7526)
  line L450 (-91.5401, 33.7526) -> (-92.2015, 33.4881)
  line L451 (-92.2015, 33.4881) -> (-92.5391, 32.5063)
  line L452 (-92.5391, 32.5063) -> (-92.5855, 31.5617)
  line L453 (-92.5855, 31.5617) -> (-92.3407, 30.6542)
  line L454 (-92.3407, 30.6542) -> (-91.8046, 29.7839)
  line L455 (-91.8046, 29.7839) -> (-92.2959, 29.0747)
  line L456 (-92.2959, 29.0747) -> (-92.8566, 28.7721)
  line L457 (-92.8566, 28.7721) -> (-93.4865, 28.8762)
  line L458 (-93.4865, 28.8762) -> (-94.1859, 29.387)
  line L459 (-94.1859, 29.387) -> (-95.5088, 29.5193)
  line L460 (-95.5088, 29.5193) -> (-94.7873, 31.4902)
  line L461 (-94.7873, 31.4902) -> (-93.5244, 33.2235)
  line L462 (-93.5244, 33.2235) -> (-92.3338, 35.8693)
  line L463 (-92.3338, 35.8693) -> (-92.5984, 36.5308)
  line L464 (-92.5984, 36.5308) -> (-93.3437, 36.7396)
  line L465 (-93.3437, 36.7396) -> (-93.9009, 37.14)
  line L466 (-93.9009, 37.14) -> (-94.2698, 37.7318)
  line L467 (-94.2698, 37.7318) -> (-94.4505, 38.5152)
  line L468 (-94.4505, 38.5152) -> (-94.9964, 38.7468)
  line L469 (-94.9964, 38.7468) -> (-95.421, 39.0886)
  line L470 (-95.421, 39.0886) -> (-95.7241, 39.5406)
  line L471 (-95.7241, 39.5406) -> (-95.9057, 40.1027)
  line L472 (-95.9057, 40.1027) -> (-95.9305, 42.5008)
  line L473 (-95.9305, 42.5008) -> (-95.5088, 44.8651)
  line L474 (-95.5088, 44.8651) -> (-95.6326, 46.2137)
  line L475 (-95.6326, 46.2137) -> (-95.9164, 46.7073)
  line L476 (-95.9164, 46.7073) -> (-96.3602, 46.3459)
  line L477 (-96.3602, 46.3459) -> (-96.964, 45.1297)
  line L478 (-96.964, 45.1297) -> (-97.0963, 44.0714)
  line L479 (-97.0963, 44.0714) -> (-96.6734, 39.317)
  line L480 (-96.6734, 39.317) -> (-96.6994, 34.5464)
  line L481 (-96.6994, 34.5464) -> (-97.0519, 33.1796)
  line L482 (-97.0519, 33.1796) -> (-97.6104, 31.9302)
  line L483 (-97.6104, 31.9302) -> (-98.3749, 30.7983)
  line L484 (-98.3749, 30.7983) -> (-99.3453, 29.7839)
  line L485 (-99.3453, 29.7839) -> (-99.4775, 28.7256)
  line L486 (-99.4775, 28.7256) -> (-100.4689, 28.6112)
  line L487 (-100.4689, 28.6112) -> (-101.1962, 28.1983)
  line L488 (-101.1962, 28.1983) -> (-101.6595, 27.4868)
  line L489 (-101.6595, 27.4868) -> (-101.8588, 26.4766)
  line L490 (-101.8588, 26.4766) -> (-101.5085, 25.7532)
  line L491 (-101.5085, 25.7532) -> (-100.9948, 25.2475)
  line L492 (-100.9948, 25.2475) -> (-100.3178, 24.9595)
  line L493 (-100.3178, 24.9595) -> (-99.4775, 24.8891)
  line L494 (-99.4775, 24.8891) -> (-98.9484, 23.9631)
  line L495 (-98.9484, 23.9631) -> (-102.2557, 19.7298)
  line L496 (-102.2557, 19.7298) -> (-102.8401, 18.6581)
  line L497 (-102.8401, 18.6581) -> (-102.8806, 18.0805)
  line L498 (-102.8806, 18.0805) -> (-102.3771, 17.9967)
  line L499 (-102.3771, 17.9967) -> (-101.3296, 18.4068)
  line L500 (-101.3296, 18.4068) -> (-98.2869, 21.8464)
  line L501 (-98.2869, 21.8464) -> (-97.8383, 21.6627)
  line L502 (-97.8383, 21.6627) -> (-97.4932, 21.3173)
  line L503 (-97.4932, 21.3173) -> (-96.6949, 19.1872)
  line L504 (-96.6949, 19.1872) -> (-96.3025, 16.9516)
  line L505 (-96.3025, 16.9516) -> (-96.5671, 15.3641)
  line L506 (-96.5671, 15.3641) -> (-98.8161, 14.9673)
  line L507 (-98.8161, 14.9673) -> (-99.1884, 14.2025)
  line L508 (-99.1884, 14.2025) -> (-99.3346, 13.4405)
  line L509 (-99.3346, 13.4405) -> (-99.2546, 12.6812)
  line L510 (-99.2546, 12.6812) -> (-98.9484, 11.9246)
  line L511 (-98.9484, 11.9246) -> (-100.139, 9.411)
  line L512 (-100.139, 9.411) -> (-100.7818, 9.0471)
  line L513 (-100.7818, 9.0471) -> (-101.437, 8.9258)
  line L514 (-101.437, 8.9258) -> (-102.1047, 9.0471)
  line L515 (-102.1047, 9.0471) -> (-102.7848, 9.411)
  line L516 (-102.7848, 9.411) -> (-103.2335, 9.2273)
  line L517 (-103.2335, 9.2273) -> (-103.5786, 8.8819)
  line L518 (-103.5786, 8.8819) -> (-104.2976, 10.5739)
  line L519 (-104.2976, 10.5739) -> (-104.6369, 12.3214)
  line L520 (-104.6369, 12.3214) -> (-104.2218, 13.5686)
  line L521 (-104.2218, 13.5686) -> (-103.5786, 14.7027)
  line L522 (-103.5786, 14.7027) -> (-103.1817, 17.6131)
  line L523 (-103.1817, 17.6131) -> (-103.9753, 18.1191)
  line L524 (-103.9753, 18.1191) -> (-104.9015, 18.4068)
  line L525 (-104.9015, 18.4068) -> (-104.8328, 19.4115)
  line L526 (-104.8328, 19.4115) -> (-104.5046, 20.3912)
  line L527 (-104.5046, 20.3912) -> (-105.4307, 22.3756)
  line L528 (-105.4307, 22.3756) -> (-105.7938, 21.6245)
  line L529 (-105.7938, 21.6245) -> (-105.9598, 20.7881)
  line L530 (-105.9598, 20.7881) -> (-106.6213, 20.5235)
  line L531 (-106.6213, 20.5235) -> (-107.5473, 20.788)
  line L532 (-107.5473, 20.788) -> (-108.4734, 20.5235)
  line L533 (-108.4734, 20.5235) -> (-109.6324, 21.0207)
  line L534 (-109.6324, 21.0207) -> (-110.59, 21.8464)
  line L535 (-110.59, 21.8464) -> (-111.3877, 21.13)
  line L536 (-111.3877, 21.13) -> (-111.6316, 20.4502)
  line L537 (-111.6316, 20.4502) -> (-111.3216, 19.8071)
  line L538 (-111.3216, 19.8071) -> (-110.4577, 19.2006)
  line L539 (-110.4577, 19.2006) -> (-110.4396, 18.5506)
  line L540 (-110.4396, 18.5506) -> (-110.61, 17.9811)
  line L541 (-110.61, 17.9811) -> (-110.9688, 17.4923)
  line L542 (-110.9688, 17.4923) -> (-111.5161, 17.0839)
  line L543 (-111.5161, 17.0839) -> (-112.135, 14.5211)
  line L544 (-112.135, 14.5211) -> (-113.1036, 12.0569)
  line L545 (-113.1036, 12.0569) -> (-114.1747, 11.5914)
  line L546 (-114.1747, 11.5914) -> (-115.3525, 11.5277)
  line L547 (-115.3525, 11.5277) -> (-115.0879, 13.6444)
  line L548 (-115.0879, 13.6444) -> (-115.8052, 13.4152)
  line L549 (-115.8052, 13.4152) -> (-116.3971, 13.4931)
  line L550 (-116.3971, 13.4931) -> (-116.8636, 13.8782)
  line L551 (-116.8636, 13.8782) -> (-117.2046, 14.5704)
  line L552 (-117.2046, 14.5704) -> (-116.7729, 16.6036)
  line L553 (-116.7729, 16.6036) -> (-116.5431, 18.6714)
  line L554 (-116.5431, 18.6714) -> (-116.1414, 19.7622)
  line L555 (-116.1414, 19.7622) -> (-115.5886, 20.28)
  line L556 (-115.5886, 20.28) -> (-114.8847, 20.2251)
  line L557 (-114.8847, 20.2251) -> (-114.0296, 19.5975)
  line L558 (-114.0296, 19.5975) -> (-112.9713, 19.4652)
  line L559 (-112.9713, 19.4652) -> (-112.9306, 21.1945)
  line L560 (-112.9306, 21.1945) -> (-112.7067, 22.9048)
  line L561 (-112.7067, 22.9048) -> (-113.7529, 22.5242)
  line L562 (-113.7529, 22.5242) -> (-114.5588, 21.7141)
  line L563 (-114.5588, 21.7141) -> (-114.9557, 21.5818)
  line L564 (-114.9557, 21.5818) -> (-115.3525, 21.7141)
  line L565 (-115.3525, 21.7141) -> (-116.0794, 22.4002)
  line L566 (-116.0794, 22.4002) -> (-116.5643, 23.1802)
  line L567 (-116.5643, 23.1802) -> (-116.807, 24.0539)
  line L568 (-116.807, 24.0539) -> (-116.8077, 25.0214)
  line L569 (-116.8077, 25.0214) -> (-114.266, 26.1329)
  line L570 (-114.266, 26.1329) -> (-111.6484, 27.0058)
  line L571 (-111.6484, 27.0058) -> (-110.5527, 28.1004)
  line L572 (-110.5527, 28.1004) -> (-109.3055, 28.9063)
  line L573 (-109.3055, 28.9063) -> (-107.9069, 29.4233)
  line L574 (-107.9069, 29.4233) -> (-106.3567, 29.6516)
  line L575 (-106.3567, 29.6516) -> (-105.6925, 30.3846)
  line L576 (-105.6925, 30.3846) -> (-105.5593, 30.8274)
  line L577 (-105.5593, 30.8274) -> (-105.957, 30.9799)
  line L578 (-105.957, 30.9799) -> (-106.8859, 30.8423)
  line L579 (-106.8859, 30.8423) -> (-108.3411, 31.636)
  line L580 (-108.3411, 31.636) -> (-112.7666, 28.8275)
  line L581 (-112.7666, 28.8275) -> (-117.4692, 26.4766)
  line L582 (-117.4692, 26.4766) -> (-118.8833, 25.3751)
  line L583 (-118.8833, 25.3751) -> (-120.115, 24.0954)
  line L584 (-120.115, 24.0954) -> (-121.2532, 24.2083)
  line L585 (-121.2532, 24.2083) -> (-122.0074, 24.6649)
  line L586 (-122.0074, 24.6649) -> (-122.3777, 25.4651)
  line L587 (-122.3777, 25.4651) -> (-122.364, 26.6089)
  line L588 (-122.364, 26.6089) -> (-120.4424, 29.6571)
  line L589 (-120.4424, 29.6571) -> (-118.9244, 32.9589)
  line L590 (-118.9244, 32.9589) -> (-114.0296, 40.4995)
  line L591 (-114.0296, 40.4995) -> (-110.9751, 42.424)
  line L592 (-110.9751, 42.424) -> (-107.6796, 43.9391)
  line L593 (-107.6796, 43.9391) -> (-105.6681, 43.9796)
  line L594 (-105.6681, 43.9796) -> (-103.7109, 43.6745)
  line L595 (-103.7109, 43.6745) -> (-103.2428, 44.2091)
  line L596 (-103.2428, 44.2091) -> (-103.2606, 44.522)
  line L597 (-103.2606, 44.522) -> (-103.4463, 44.8651)
  line L598 (-103.4463, 44.8651) -> (-105.0338, 45.7912)
  line L599 (-105.0338, 45.7912) -> (-105.7761, 46.6797)
  line L600 (-105.7761, 46.6797) -> (-106.0774, 46.8605)
  line L601 (-106.0774, 46.8605) -> (-106.3322, 46.8657)
  line L602 (-106.3322, 46.8657) -> (-106.7021, 46.349)
  line L603 (-106.7021, 46.349) -> (-106.8859, 45.1297)
  line L604 (-106.8859, 45.1297) -> (-114.2942, 42.8808)
  line L605 (-114.2942, 42.8808) -> (-116.3447, 41.0948)
  line L606 (-116.3447, 41.0948) -> (-118.1306, 39.0443)
  line L607 (-118.1306, 39.0443) -> (-119.3213, 35.3402)
  line L608 (-119.3213, 35.3402) -> (-121.2131, 32.8805)
  line L609 (-121.2131, 32.8805) -> (-122.7609, 30.1808)
  line L610 (-122.7609, 30.1808) -> (-124.6129, 29.7839)
  line L611 (-124.6129, 29.7839) -> (-124.935, 28.9483)
  line L612 (-124.935, 28.9483) -> (-125.4067, 28.1964)
  line L613 (-125.4067, 28.1964) -> (-126.3327, 29.2548)
  line L614 (-126.3327, 29.2548) -> (-126.8503, 28.4975)
  line L615 (-126.8503, 28.4975) -> (-126.8619, 27.6673)
  line L616 (-126.8619, 27.6673) -> (-127.9352, 28.4335)
  line L617 (-127.9352, 28.4335) -> (-129.2431, 28.7256)
  line L618 (-129.2431, 28.7256) -> (-130.8682, 28.2741)
  line L619 (-130.8682, 28.2741) -> (-132.5504, 28.0641)
  line L620 (-132.5504, 28.0641) -> (-134.1379, 26.6089)
  line L621 (-134.1379, 26.6089) -> (-134.7994, 27.1381)
  line L622 (-134.7994, 27.1381) -> (-135.7254, 33.6204)
  line L623 (-135.7254, 33.6204) -> (-135.064, 35.8693)
  line L624 (-135.064, 35.8693) -> (-133.952, 36.6817)
  line L625 (-133.952, 36.6817) -> (-133.0302, 37.636)
  line L626 (-133.0302, 37.636) -> (-132.2984, 38.7322)
  line L627 (-132.2984, 38.7322) -> (-131.7567, 39.9704)
  line L628 (-131.7567, 39.9704) -> (-131.889, 43.8068)
  line L629 (-131.889, 43.8068) -> (-132.4181, 45.9235)
  line L630 (-132.4181, 45.9235) -> (-134.113, 48.7901)
  line L631 (-134.113, 48.7901) -> (-135.99, 51.4797)
  line L632 (-135.99, 51.4797) -> (-138.1067, 50.686)
  line L633 (-138.1067, 50.686) -> (-138.1067, 105.9838)
  line L634 (-6.8735, 98.0463) -> (-6.6625, 98.2828)
  line L635 (-6.6625, 98.2828) -> (-6.3443, 98.1786)
  line L636 (-6.3443, 98.1786) -> (-5.1537, 96.988)
  line L637 (-5.1537, 96.988) -> (-5.0381, 96.5643)
  line L638 (-5.0381, 96.5643) -> (-5.286, 96.1943)
  line L639 (-5.286, 96.1943) -> (-6.2224, 97.0158)
  line L640 (-6.2224, 97.0158) -> (-6.8735, 98.0463)
  line L641 (23.8181, 34.811) -> (23.8181, 31.9006)
  line L642 (23.8181, 31.9006) -> (22.6367, 32.02)
  line L643 (22.6367, 32.02) -> (21.5594, 32.3685)
  line L644 (21.5594, 32.3685) -> (20.5861, 32.9461)
  line L645 (20.5861, 32.9461) -> (19.7171, 33.7527)
  line L646 (19.7171, 33.7527) -> (18.9426, 36.0792)
  line L647 (18.9426, 36.0792) -> (17.865, 38.2506)
  line L648 (17.865, 38.2506) -> (17.0713, 35.0756)
  line L649 (17.0713, 35.0756) -> (15.9392, 36.2073)
  line L650 (15.9392, 36.2073) -> (14.9546, 37.4568)
  line L651 (14.9546, 37.4568) -> (13.4169, 41.5405)
  line L652 (13.4169, 41.5405) -> (12.4411, 45.7912)
  line L653 (12.4411, 45.7912) -> (13.4826, 47.89)
  line L654 (13.4826, 47.89) -> (14.69, 49.8922)
  line L655 (14.69, 49.8922) -> (14.8224, 50.686)
  line L656 (14.8224, 50.686) -> (14.69, 51.4797)
  line L657 (14.69, 51.4797) -> (14.0409, 51.8708)
  line L658 (14.0409, 51.8708) -> (13.4994, 52.4058)
  line L659 (13.4994, 52.4058) -> (13.1025, 52.5381)
  line L660 (13.1025, 52.5381) -> (12.7056, 52.4058)
  line L661 (12.7056, 52.4058) -> (12.0236, 51.101)
  line L662 (12.0236, 51.101) -> (11.7796, 49.6276)
  line L663 (11.7796, 49.6276) -> (11.1249, 49.1663)
  line L664 (11.1249, 49.1663) -> (10.3244, 49.2308)
  line L665 (10.3244, 49.2308) -> (9.6544, 49.9011)
  line L666 (9.6544, 49.9011) -> (8.8692, 50.4214)
  line L667 (8.8692, 50.4214) -> (8.34, 52.8026)
  line L668 (8.34, 52.8026) -> (7.1968, 54.474)
  line L669 (7.1968, 54.474) -> (6.2234, 56.2422)
  line L670 (6.2234, 56.2422) -> (6.2148, 57.2681)
  line L671 (6.2148, 57.2681) -> (6.6202, 58.2266)
  line L672 (6.6202, 58.2266) -> (6.2596, 59.0815)
  line L673 (6.2596, 59.0815) -> (5.5619, 59.6818)
  line L674 (5.5619, 59.6818) -> (4.1067, 56.2422)
  line L675 (4.1067, 56.2422) -> (3.667, 56.0073)
  line L676 (3.667, 56.0073) -> (3.1807, 56.1099)
  line L677 (3.1807, 56.1099) -> (1.064, 58.3589)
  line L678 (1.064, 58.3589) -> (2.7838, 59.4172)
  line L679 (2.7838, 59.4172) -> (2.7802, 59.9612)
  line L680 (2.7802, 59.9612) -> (2.5192, 60.4755)
  line L681 (2.5192, 60.4755) -> (1.4363, 61.0117)
  line L682 (1.4363, 61.0117) -> (0.2702, 61.4016)
  line L683 (0.2702, 61.4016) -> (-0.2869, 62.2233)
  line L684 (-0.2869, 62.2233) -> (-1.0527, 62.8568)
  line L685 (-1.0527, 62.8568) -> (-1.5099, 62.4174)
  line L686 (-1.5099, 62.4174) -> (-1.7141, 61.7985)
  line L687 (-1.7141, 61.7985) -> (-1.9519, 60.5517)
  line L688 (-1.9519, 60.5517) -> (-1.7004, 59.651)
  line L689 (-1.7004, 59.651) -> (-0.9597, 59.0965)
  line L690 (-0.9597, 59.0965) -> (0.2702, 58.888)
  line L691 (0.2702, 58.888) -> (-0.794, 58.2255)
  line L692 (-0.794, 58.2255) -> (-1.9787, 57.8297)
  line L693 (-1.9787, 57.8297) -> (-1.9988, 54.8951)
  line L694 (-1.9988, 54.8951) -> (-1.4495, 52.0089)
  line L695 (-1.4495, 52.0089) -> (-0.7881, 51.3474)
  line L696 (-0.7881, 51.3474) -> (1.5932, 50.4214)
  line L697 (1.5932, 50.4214) -> (0.1388, 49.1654)
  line L698 (0.1388, 49.1654) -> (-1.185, 47.7756)
  line L699 (-1.185, 47.7756) -> (-1.5818, 45.262)
  line L700 (-1.5818, 45.262) -> (-0.5235, 43.5422)
  line L701 (-0.5235, 43.5422) -> (-1.1585, 42.2753)
  line L702 (-1.1585, 42.2753) -> (-1.304, 41.0592)
  line L703 (-1.304, 41.0592) -> (-0.96, 39.894)
  line L704 (-0.96, 39.894) -> (-0.1266, 38.7797)
  line L705 (-0.1266, 38.7797) -> (1.7255, 34.2818)
  line L706 (1.7255, 34.2818) -> (1.064, 30.3131)
  line L707 (1.064, 30.3131) -> (1.99, 24.2277)
  line L708 (1.99, 24.2277) -> (2.5192, 23.6985)
  line L709 (2.5192, 23.6985) -> (2.7443, 24.3377)
  line L710 (2.7443, 24.3377) -> (3.1059, 24.8153)
  line L711 (3.1059, 24.8153) -> (3.6042, 25.1314)
  line L712 (3.6042, 25.1314) -> (4.239, 25.286)
  line L713 (4.239, 25.286) -> (4.0622, 24.4023)
  line L714 (4.0622, 24.4023) -> (3.7098, 23.5662)
  line L715 (3.7098, 23.5662) -> (4.0854, 22.9998)
  line L716 (4.0854, 22.9998) -> (4.7682, 23.0371)
  line L717 (4.7682, 23.0371) -> (5.8265, 26.4766)
  line L718 (5.8265, 26.4766) -> (4.9502, 28.0407)
  line L719 (4.9502, 28.0407) -> (4.3713, 29.7839)
  line L720 (4.3713, 29.7839) -> (4.3413, 30.3876)
  line L721 (4.3413, 30.3876) -> (4.4636, 30.9416)
  line L722 (4.4636, 30.9416) -> (4.7381, 31.4459)
  line L723 (4.7381, 31.4459) -> (5.165, 31.9006)
  line L724 (5.165, 31.9006) -> (6.0366, 30.7639)
  line L725 (6.0366, 30.7639) -> (6.7525, 29.5193)
  line L726 (6.7525, 29.5193) -> (7.0286, 30.5893)
  line L727 (7.0286, 30.5893) -> (7.8109, 31.3714)
  line L728 (7.8109, 31.3714) -> (8.8807, 29.2136)
  line L729 (8.8807, 29.2136) -> (9.5306, 26.8735)
  line L730 (9.5306, 26.8735) -> (8.0754, 17.6131)
  line L731 (8.0754, 17.6131) -> (8.3833, 17.3914)
  line L732 (8.3833, 17.3914) -> (8.7369, 17.4808)
  line L733 (8.7369, 17.4808) -> (10.1921, 19.2006)
  line L734 (10.1921, 19.2006) -> (10.7439, 18.6086)
  line L735 (10.7439, 18.6086) -> (11.1181, 17.8777)
  line L736 (11.1181, 17.8777) -> (12.0111, 18.2994)
  line L737 (12.0111, 18.2994) -> (12.9702, 18.5391)
  line L738 (12.9702, 18.5391) -> (13.0983, 18.9926)
  line L739 (13.0983, 18.9926) -> (13.0087, 19.298)
  line L740 (13.0087, 19.298) -> (12.7014, 19.4555)
  line L741 (12.7014, 19.4555) -> (12.1765, 19.4652)
  line L742 (12.1765, 19.4652) -> (12.2496, 22.1378)
  line L743 (12.2496, 22.1378) -> (12.7056, 24.7568)
  line L744 (12.7056, 24.7568) -> (12.3439, 26.9951)
  line L745 (12.3439, 26.9951) -> (12.3088, 29.2548)
  line L746 (12.3088, 29.2548) -> (12.7056, 30.0485)
  line L747 (12.7056, 30.0485) -> (13.5917, 29.6284)
  line L748 (13.5917, 29.6284) -> (14.5577, 29.6516)
  line L749 (14.5577, 29.6516) -> (14.4795, 31.3956)
  line L750 (14.4795, 31.3956) -> (13.9684, 32.925)
  line L751 (13.9684, 32.925) -> (13.0243, 34.2399)
  line L752 (13.0243, 34.2399) -> (11.6473, 35.3402)
  line L753 (11.6473, 35.3402) -> (11.3277, 36.2706)
  line L754 (11.3277, 36.2706) -> (10.9346, 36.6249)
  line L755 (10.9346, 36.6249) -> (10.4678, 36.4029)
  line L756 (10.4678, 36.4029) -> (9.9275, 35.6047)
  line L757 (9.9275, 35.6047) -> (9.921, 34.5656)
  line L758 (9.921, 34.5656) -> (9.6322, 33.69)
  line L759 (9.6322, 33.69) -> (9.0611, 32.9781)
  line L760 (9.0611, 32.9781) -> (8.2077, 32.4297)
  line L761 (8.2077, 32.4297) -> (7.6786, 33.0912)
  line L762 (7.6786, 33.0912) -> (8.3656, 34.6652)
  line L763 (8.3656, 34.6652) -> (8.4723, 36.3985)
  line L764 (8.4723, 36.3985) -> (8.1489, 39.2799)
  line L765 (8.1489, 39.2799) -> (7.414, 42.087)
  line L766 (7.414, 42.087) -> (7.539, 42.4625)
  line L767 (7.539, 42.4625) -> (7.8109, 42.7485)
  line L768 (7.8109, 42.7485) -> (9.1338, 41.9547)
  line L769 (9.1338, 41.9547) -> (9.7952, 42.2193)
  line L770 (9.7952, 42.2193) -> (10.4567, 41.9547)
  line L771 (10.4567, 41.9547) -> (10.3309, 40.9062)
  line L772 (10.3309, 40.9062) -> (9.7952, 39.9704)
  line L773 (9.7952, 39.9704) -> (10.0598, 39.3089)
  line L774 (10.0598, 39.3089) -> (10.9169, 39.1859)
  line L775 (10.9169, 39.1859) -> (11.7097, 38.8803)
  line L776 (11.7097, 38.8803) -> (12.4382, 38.3921)
  line L777 (12.4382, 38.3921) -> (13.1025, 37.7214)
  line L778 (13.1025, 37.7214) -> (13.6792, 36.6144)
  line L779 (13.6792, 36.6144) -> (14.4254, 35.6047)
  line L780 (14.4254, 35.6047) -> (14.9546, 33.2235)
  line L781 (14.9546, 33.2235) -> (15.8599, 32.5483)
  line L782 (15.8599, 32.5483) -> (16.5806, 32.4555)
  line L783 (16.5806, 32.4555) -> (17.1167, 32.9452)
  line L784 (17.1167, 32.9452) -> (17.4681, 34.0172)
  line L785 (17.4681, 34.0172) -> (18.6588, 30.8423)
  line L786 (18.6588, 30.8423) -> (20.7754, 29.7839)
  line L787 (20.7754, 29.7839) -> (21.1604, 28.3645)
  line L788 (21.1604, 28.3645) -> (21.7015, 27.0058)
  line L789 (21.7015, 27.0058) -> (21.3562, 26.4476)
  line L790 (21.3562, 26.4476) -> (21.1723, 25.8152)
  line L791 (21.1723, 25.8152) -> (21.4309, 24.9688)
  line L792 (21.4309, 24.9688) -> (21.3627, 24.2457)
  line L793 (21.3627, 24.2457) -> (20.9679, 23.6459)
  line L794 (20.9679, 23.6459) -> (20.2463, 23.1693)
  line L795 (20.2463, 23.1693) -> (20.114, 21.8464)
  line L796 (20.114, 21.8464) -> (19.2521, 21.8647)
  line L797 (19.2521, 21.8647) -> (18.6121, 22.1574)
  line L798 (18.6121, 22.1574) -> (18.1939, 22.7246)
  line L799 (18.1939, 22.7246) -> (17.9973, 23.5662)
  line L800 (17.9973, 23.5662) -> (17.4681, 23.6986)
  line L801 (17.4681, 23.6986) -> (16.939, 23.5662)
  line L802 (16.939, 23.5662) -> (15.9581, 22.6793)
  line L803 (15.9581, 22.6793) -> (15.2564, 21.6561)
  line L804 (15.2564, 21.6561) -> (14.8337, 20.4965)
  line L805 (14.8337, 20.4965) -> (14.69, 19.2006)
  line L806 (14.69, 19.2006) -> (13.2348, 15.4964)
  line L807 (13.2348, 15.4964) -> (14.1321, 15.4049)
  line L808 (14.1321, 15.4049) -> (14.8223, 14.835)
  line L809 (14.8223, 14.835) -> (14.3741, 14.3983)
  line L810 (14.3741, 14.3983) -> (13.894, 14.2307)
  line L811 (13.894, 14.2307) -> (13.382, 14.3322)
  line L812 (13.382, 14.3322) -> (12.8379, 14.7027)
  line L813 (12.8379, 14.7027) -> (12.3893, 14.519)
  line L814 (12.3893, 14.519) -> (12.0442, 14.1735)
  line L815 (12.0442, 14.1735) -> (11.2504, 6.236)
  line L816 (11.2504, 6.236) -> (10.0246, 5.2733)
  line L817 (10.0246, 5.2733) -> (9.131, 4.1145)
  line L818 (9.131, 4.1145) -> (8.5694, 2.7597)
  line L819 (8.5694, 2.7597) -> (8.34, 1.209)
  line L820 (8.34, 1.209) -> (7.3492, -0.3101)
  line L821 (7.3492, -0.3101) -> (6.6202, -1.966)
  line L822 (6.6202, -1.966) -> (0.0057, -1.966)
  line L823 (0.0057, -1.966) -> (-0.3912, -1.5691)
  line L824 (-0.3912, -1.5691) -> (-0.7881, -1.4368)
  line L825 (-0.7881, -1.4368) -> (-1.185, -1.5691)
  line L826 (-1.185, -1.5691) -> (-1.5818, -1.966)
  line L827 (-1.5818, -1.966) -> (-5.8152, -1.966)
  line L828 (-5.8152, -1.966) -> (-5.9384, 0.086)
  line L829 (-5.9384, 0.086) -> (-6.6089, 2.0027)
  line L830 (-6.6089, 2.0027) -> (-7.9318, -0.5108)
  line L831 (-7.9318, -0.5108) -> (-8.6951, -0.6098)
  line L832 (-8.6951, -0.6098) -> (-9.3243, -0.4444)
  line L833 (-9.3243, -0.4444) -> (-9.8195, -0.0145)
  line L834 (-9.8195, -0.0145) -> (-10.1808, 0.6798)
  line L835 (-10.1808, 0.6798) -> (-10.7265, 1.82)
  line L836 (-10.7265, 1.82) -> (-10.9745, 3.061)
  line L837 (-10.9745, 3.061) -> (-11.0517, 5.8671)
  line L838 (-11.0517, 5.8671) -> (-10.7099, 8.6173)
  line L839 (-10.7099, 8.6173) -> (-11.1642, 9.0262)
  line L840 (-11.1642, 9.0262) -> (-11.7683, 9.1464)
  line L841 (-11.7683, 9.1464) -> (-12.6256, 8.9641)
  line L842 (-12.6256, 8.9641) -> (-13.4881, 9.0142)